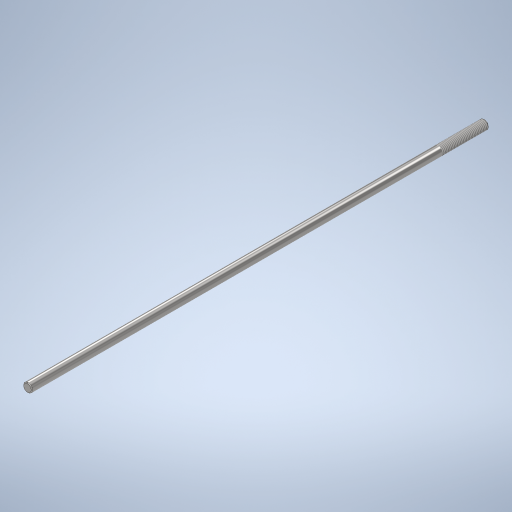
# Autodesk Inventor part: 2309HCMUTE-CDT23-TRUC_TRUOT
Saved by Autodesk Inventor 2023 (Build 270158000, 158)
## iProperties
Created: 2023-10-22
Part Number: 2309HCMUTE-CDT23-TRUC_TRUOT
Material: Stainless Steel
Document SubType Name: Modeling
Designer: havie
Density: 8 g/cm^3
Appearance: Semi-Polished
Author: havie
Autodesk Inventor part; units mm, degrees
ref_plane "YZ Plane" through (0, 0, 0) normal (1, 0, 0) x (0, 1, 0)
ref_plane "XZ Plane" through (0, 0, 0) normal (0, 1, 0) x (-1, 0, 0)
ref_plane "XY Plane" through (0, 0, 0) normal (0, 0, 1) x (1, 0, 0)
sketch "Sketch1" plane through (0, 0, 0) normal (0, 1, 0) x (-1, 0, 0)
  circle A0 centre (0, 0) radius 3
  dimension "d0" = 6
  constraints: 1 centre point, 1 coincident
  measures "d0" diameter of A0
extrude "Extrusion1" add sketch "Sketch1" along normal blind 300
fillet "Fillet1" radius 0.5 2 edges at (3, 300, 0) (3, 0, 0)
thread "Thread1" size "M6x1" class "6g" standard "ISO Metric profile" length 30
body "Solid1"
